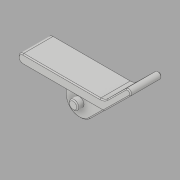
# Autodesk Inventor part: Ejector
Saved by Autodesk Inventor 2019.4 (Build 234330000, 330)
## iProperties
Created: 2021-10-02
Part Number: Ejector
Material: Generic
Document SubType Name: Modeling
Designer: erics
Mass: 0.77284 g
Surface Area: 8.51521 cm^2
Volume: 0.77284 cm^3
Density: 1 g/cm^3
Appearance: Default
Author: erics
Autodesk Inventor part; units mm, degrees
ref_plane "YZ Plane" through (0, 0, 0) normal (1, 0, 0) x (0, 1, 0)
ref_plane "XZ Plane" through (0, 0, 0) normal (0, 1, 0) x (-1, 0, 0)
ref_plane "XY Plane" through (0, 0, 0) normal (0, 0, 1) x (1, 0, 0)
sketch "Sketch1" plane through (0, 0, 0) normal (0, 0, 1) x (1, 0, 0)
  line L0 (-10.16, 8.73125) -> (10.625192, 8.73125)
  line L1 (12.409746, 9.463774) -> (17.628413, 14.616259)
  line L2 (17.628413, 14.616259) -> (18.743759, 13.486587) construction
  line L3 (18.743759, 13.486587) -> (1.466185, -3.571875)
  line L4 (1.466185, -3.571875) -> (-3.571875, -3.571875) construction
  line L5 (-3.571875, -3.571875) -> (-3.571875, 0) construction
  line L6 (-6.111875, 6.35) -> (-10.16, 6.35)
  line L7 (-10.16, 6.35) -> (-10.16, 8.73125) construction
  circle A0 centre (0, 0) radius 1.1811
  arc A1 (-8.969375, 8.73125) -> (-8.969375, 6.35) centre (-8.969375, 7.540625) ccw
  arc A2 (18.178923, 12.928914) -> (17.063577, 14.058586) centre (17.62125, 13.49375) ccw
  arc A3 (-3.571875, 0) -> (2.509528, -2.541763) centre (0, 0) ccw
  arc A4 (-3.571875, 3.81) -> (-6.111875, 6.35) centre (-6.111875, 3.81) ccw
  arc A5 (10.625192, 8.73125) -> (12.409746, 9.463774) centre (10.625192, 11.27125) ccw
  line L8 (-3.571875, 0) -> (-3.571875, 3.81)
  line L9 (-6.111875, 6.35) -> (11.515504, 6.35)
  dimension "d0" = 10.16
  dimension "d1" = 6.35
  dimension "d2" = 1.5875
  dimension "d3" = 7.9375
  dimension "d5" = 2.3622
  dimension "d6" = 28.575
  dimension "d10" = 17.85938
  dimension "d12" = 2.38125
  dimension "d13" = 2.54
  dimension "d14" = 2.54
  constraints: 20 end point, 15 tangent, 10 point on circle, 6 centre point, 6 perpendicular, 6 point on line, 2 coincident, 2 horizontal, 2 parallel
  measures "d0" distance from line of A0.centre L7
  measures "d1" distance from line of A0.centre L6
  measures "d2" distance between parallel lines of L3 L1
  measures "d5" diameter of A0
  measures "d12" distance of L6.end L0.start
  measures "d13" radius of A5
  measures "d14" radius of A4
extrude "Extrusion1" add sketch "Sketch1" against normal blind 2.54 contours L0 A5 L1 A2 L3 L9 L6 A1 | L9 L3 A3 L8 A4 | A0
extrude "Extrusion2" add sketch "Sketch1" along normal blind 1.5875 contours A0
extrude "Extrusion3" add sketch "Sketch1" along normal blind 5.3975 contours L0 A5 L1 A2 L3 L9 L6 A1
chamfer "Chamfer1" distance 0.254 angle 45 22 edges at (-1.1811, 0, 1.5875) (0.8279, 8.7312, 5.3975) (-10.16, 7.5406, 5.3975) (1.2731, 6.35, 5.3975) (11.5897, 8.9215, 5.3975) (14.7367, 11.7612, 5.3975) (18.1861, 14.0514, 5.3975) (14.8472, 9.6395, 5.3975) (0.8279, 8.7312, -2.54) (11.5897, 8.9215, -2.54) (14.7367, 11.7612, -2.54) (18.1861, 14.0514, -2.54) (10.3442, 5.1936, -2.54) (-1.3774, -3.2956, -2.54) (-3.5719, 1.905, -2.54) (-4.3158, 5.6061, -2.54) (-7.5406, 6.35, -2.54) (-10.16, 7.5406, -2.54) (-3.5719, 1.905, 0) (-4.3158, 5.6061, 0) (-1.3774, -3.2956, 0) (7.0125, 1.9041, 0)
body "Solid1"
